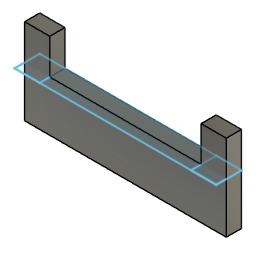
MicroMouse_BatteryHolding v3 (Autodesk Fusion 360 design; units mm, degrees)
Autodesk Fusion 360 part; units mm, degrees
sketch "Sketch1" plane through (0, 0, 0) normal (0, 0, 1) x (1, 0, 0)
  line L0 (-75, 25) -> (-35, 25)
  line L1 (-35, 25) -> (-35, 20)
  line L2 (-35, 20) -> (-75, 20)
  line L3 (-75, 20) -> (-75, 25)
  line L4 (-75, 20) -> (-70, 20)
  line L5 (-70, 20) -> (-70, 25)
  line L6 (-70, 25) -> (-75, 25)
  line L7 (-75, 25) -> (-75, 20)
  line L8 (-40, 20) -> (-35, 20)
  line L9 (-35, 20) -> (-35, 25)
  line L10 (-35, 25) -> (-40, 25)
  line L11 (-40, 25) -> (-40, 20)
  dimension "d1" = 40
  dimension "d2" = 5
  constraint horizontal L0
  constraint vertical L1
  constraint horizontal L2
  constraint vertical L3
  constraint horizontal L4
  constraint vertical L5
  constraint horizontal L6
  constraint vertical L7
  constraint coincident L0 L5.end
  constraint horizontal L8
  constraint vertical L9
  constraint horizontal L10
  constraint vertical L11
  measures "d1" distance of L0.start L0.end
  measures "d2" distance of L0.start L2.end
extrude "Extrude1" add sketch "Sketch1" along normal blind 7 contours L0 L2 L3 L4 L5 L6 L7 | L0 L1 L2 L8 L9 L10 L11 makes body 1 at (-70, 21.6667, 2.3333) makes body 2 at (-38.3333, 25, 2.3333)
extrude "Extrude2" add sketch "Sketch1" against normal blind 8 bodies 1 2
extrude "Extrude3" add 1 faces at (-61.6667, 21.6667, -8) along direction (0, 0, -1) blind 2 on bodies 1 bodies 1
extrude "Extrude4" cut 1 faces at (-50, 20, -6.6667) along direction (0, 1, 0) blind 2 on bodies 1 bodies 1
sketch "Sketch2" plane through (0, 25, 0) normal (0, 1, 0) x (-1, 0, 0)
  line L0 (75, -10) -> (75, 7)
  line L1 (75, 7) -> (70, 7)
  line L2 (70, 7) -> (70, 0)
  line L3 (70, 0) -> (40, 0)
  line L4 (40, 0) -> (40, 7)
  line L5 (40, 7) -> (35, 7)
  line L6 (35, 7) -> (35, -10)
  line L7 (35, -10) -> (75, -10)
